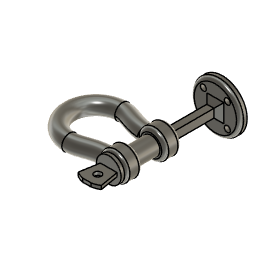
shackle v8 (Autodesk Fusion 360 design; units mm, degrees)
Autodesk Fusion 360 part; units mm, degrees
note: some values were not read from the file. Set by a fixed rule: which sketch regions a step uses.
sketch "Sketch1" plane through (0, 0, 0) normal (0, 0, 1) x (1, 0, 0)
  line L0 (0, 0) -> (0, -150) construction
  circle A0 centre (-62, -27) radius 37.5 construction
  line L1 (-62, -27) -> (-24.5, -27) construction
  line L2 (-62, -27) -> (-62, 10.5) construction
  spline S0 degree 5 poles (-62, 10.5) (-60.8613, 10.5) (-58.5805, 10.3966) (-55.1495, 9.9312) (-50.5421, 8.7566) (-44.6616, 6.7239) (-38.5882, 4.5603) (-32.2745, 2.6688) (-25.7346, 1.3084) (-19.0751, 0.4971) (-12.4478, 0.1204) (-7.3007, 0.0282) (-3.5865, 0.0051) (-1.1833, 0) (0, 0) knots 0 0 0 0 0 0 0.1 0.2 0.3 0.4 0.5 0.6 0.7 0.8 0.9 1 1 1 1 1 1
  line L3 (-6, 0) -> (6, 0)
  line L4 (-68, 10.5) -> (-56, 10.5)
  spline S1 degree 5 poles (-62, -64.5) (-60.8613, -64.5) (-58.5805, -64.3966) (-55.1495, -63.9312) (-50.5421, -62.7566) (-44.6616, -60.7239) (-38.5882, -58.5603) (-32.2745, -56.6688) (-25.7346, -55.3084) (-19.0751, -54.4971) (-12.4478, -54.1204) (-7.3007, -54.0282) (-3.5865, -54.0051) (-1.1833, -54) (0, -54) knots 0 0 0 0 0 0 0.1 0.2 0.3 0.4 0.5 0.6 0.7 0.8 0.9 1 1 1 1 1 1
  line L5 (-68, -64.5) -> (-56, -64.5)
  line L6 (-6, -54) -> (6, -54)
  arc A1 (-62, 10.5) -> (-62, -64.5) centre (-62, -27) ccw
  line L7 (-24.5, -27) -> (0, -27) construction
  line L8 (0, 0) -> (0, -27) construction
  point P0 (-33, 3)
  point P1 (-33, -57)
  dimension "d1" = 150
  dimension "d2" = 75
  constraint coincident L0.start S0.end
  constraint vertical L0
  constraint coincident A0.centre L1.start
  constraint coincident A0 L1.end
  constraint horizontal L1
  constraint coincident A0 L2.end
  constraint perpendicular L1 L2
  constraint midpoint L0.start L3
  constraint midpoint L2.end L4
  constraint tangent A0 L4
  constraint symmetric L0.start L1 S1.end
  constraint symmetric L1 L2.end S1.start
  constraint symmetric L1 P0 P1
  constraint symmetric L1 L3.start L6.start
  constraint symmetric L1 L3.end L6.end
  constraint symmetric L1 L4.start L5.start
  constraint symmetric L1 L4.end L5.end
  constraint coincident L0 L7.end
  constraint perpendicular L0 L7
  measures "d1" distance of L0.start L0.end
  measures "d2" diameter of A0
ref_plane "WorkPlane1" through (0, 0, 0) normal (1, 0, 0) x (0, 1, 0)
sketch "Sketch2" plane through (0, 0, 0) normal (1, 0, 0) x (0, 1, 0)
  circle A0 centre (0, 0) radius 11
  dimension "d4" = 22
  constraint coincident A0.centre origin
  measures "d4" diameter of A0
sweep "Sweep1" add profiles "Sketch2" path "Sketch1" along S1 A1 S0 section 1 makes body 1
sketch "Sketch3" plane through (0, 0, 0) normal (0, 1, 0) x (1, 0, 0)
  circle A0 centre (0, 0) radius 20
  circle A1 centre (0, 0) radius 12.5
  line L0 (5, -6) -> (-5, -6)
  line L1 (-5, -6) -> (-5, 6)
  line L2 (-5, 6) -> (5, 6)
  line L3 (5, 6) -> (5, -6)
  line L4 (5, -6) -> (-5, 6) construction
  line L5 (-5, -6) -> (5, 6) construction
  line L6 (-5.3, 6.3) -> (5.3, 6.3)
  line L7 (5.3, 6.3) -> (5.3, -6.3)
  line L8 (5.3, -6.3) -> (-5.3, -6.3)
  line L9 (-5.3, -6.3) -> (-5.3, 6.3)
  dimension "d11" = 40
  dimension "d16" = 25
  dimension "d70" = 10
  dimension "d71" = 12
  dimension "d72" = -0.3
  constraint coincident A0.centre A1.centre
  constraint concentric A0 A1
  constraint horizontal L0
  constraint perpendicular L0 L1
  constraint parallel L0 L2
  constraint parallel L1 L3
  constraint coincident L4 A0.centre
  constraint coincident L5 A0.centre
  measures "d11" diameter of A0
  measures "d16" diameter of A1
  measures "d70" distance of L1.end L2.end
  measures "d71" distance of L0.end L1.end
ref_plane "WorkPlane2" through (0, -27, 0) normal (0, 1, 0) x (0, 0, 1)
extrude "Extrude3" add sketch "Sketch3" along normal blind 12 and the other way blind 11 separate body contours A0 makes body 2
mirror "Mirror1" about plane through (0, -27, 0) normal (0, 1, 0) of bodies 2 makes body 3
combine "Combine1" operation add target body 1 tool bodies 2 3
extrude "Extrude4" cut sketch "Sketch3" along normal blind 16 and the other way blind 69 contours A1 | L0 L1 L2 L3 | L6 L7 L8 L9 bodies 1
fillet "Fillet1" radius 5 4 edges at (-18.6465, -43, -7.2323) (-18.6465, 12, 7.2323) (-18.6465, -11, -7.2323) (-18.6465, -66, 7.2323) on bodies 1
sketch "Sketch4" plane through (0, -66, 0) normal (0, -1, 0) x (1, 0, 0)
  circle A0 centre (0, 0) radius 12.5
  circle A1 centre (0, 0) radius 15
  circle A2 centre (0, 0) radius 12.5
  circle A3 centre (0, 0) radius 17.5
  line L0 (-17.5, 0.0312) -> (17.5, 0.0312) construction
  line L1 (17.3205, 2.5) -> (-17.3205, 2.5)
  line L2 (-17.3205, 2.5) -> (-17.3205, -2.5)
  line L3 (-17.3205, -2.5) -> (17.3205, -2.5)
  line L4 (17.3205, -2.5) -> (17.3205, 2.5)
  line L5 (17.3205, 2.5) -> (-17.3205, -2.5) construction
  line L6 (-17.3205, 2.5) -> (17.3205, -2.5) construction
  dimension "d35" = 25
  dimension "d36" = 35
  dimension "d39" = 5
  constraint coincident A0.centre A1.centre
  constraint coincident A3 L0.start
  constraint coincident A3 L0.end
  constraint horizontal L0
  constraint horizontal L1
  constraint perpendicular L1 L2
  constraint parallel L1 L3
  constraint parallel L2 L4
  constraint coincident A3 L1.start
  constraint coincident L5 A0.centre
  constraint coincident L6 A0.centre
  measures "d35" diameter of A2
  measures "d36" diameter of A3
  measures "d39" distance of L1.end L2.end
extrude "Extrude5" add sketch "Sketch4" along normal blind 5 bodies 1
extrude "Extrude6" add sketch "Sketch4" along normal blind 36 contours A0 A2 L1 L3 | A0 A1 A2 L1 L3 | A0 A1 A2 L1 L3 | A1 L1 L3 L4 | A1 L1 L2 L3 bodies 1
sketch "Sketch5" plane through (0, 0, 2.5) normal (0, 0, 1) x (-1, 0, 0)
  line L0 (-17.3205, 71) -> (17.3205, 71)
  line L1 (17.3205, 71) -> (17.3205, 102)
  line L2 (17.3205, 102) -> (-17.3205, 102)
  line L3 (-17.3205, 102) -> (-17.3205, 71)
  line L4 (0, 71) -> (0, 102) construction
  line L5 (11.7769, 71) -> (16.3887, 97.963)
  line L6 (-11.7769, 71) -> (-16.3887, 97.963)
  arc A0 (16.3887, 97.963) -> (-16.3887, 97.963) centre (0, 71.1337) ccw
  circle A1 centre (0, 86.5) radius 5
  dimension "d42" = 10
  constraint midpoint L0 L4.start
  constraint midpoint L2 L4.end
  constraint coincident L0 L5.start
  constraint symmetric L4 L5.start L6.start
  constraint symmetric L4 L5.end L6.end
  constraint midpoint L4 A1.centre
  measures "d42" diameter of A1
extrude "Extrude7" cut sketch "Sketch5" along normal up to surface (5 mm away) from surface at -5 contours L0 L2 L3 L6 A0 | L0 L1 L2 L5 A0 | A1 bodies 1
extrude "Extrude8" add sketch "Sketch3" along normal blind 12 and the other way up to surface (66 mm away) contours A1 | L0 L1 L2 L3 | L6 L7 L8 L9 bodies 1
extrude "Extrude12" cut sketch "Sketch3" along normal through all and the other way blind 40 contours L0 L1 L2 L3 | L6 L7 L8 L9 bodies 1
extrude "Extrude13" add sketch "Sketch3" along normal blind 90 and the other way blind 40 separate body contours L0 L1 L2 L3 makes body 4
sketch "Sketch8" plane through (0, 90, 0) normal (0, 1, 0) x (-1, 0, 0)
  line L0 (-5, -6) -> (5, -6)
  line L1 (5, -6) -> (5, 6)
  line L2 (5, 6) -> (-5, 6)
  line L3 (-5, 6) -> (-5, -6)
  circle A0 centre (0, 0) radius 35
  circle A1 centre (0, 0) radius 24 construction
  line L4 (0, 0) -> (24.7487, 24.7487) construction
  line L5 (0, 0) -> (35, 0) construction
  circle A2 centre (16.9706, 16.9706) radius 4.25
  circle A3 centre (-16.9706, 16.9706) radius 4.25
  circle A4 centre (-16.9706, -16.9706) radius 4.25
  circle A5 centre (16.9706, -16.9706) radius 4.25
  circle A6 centre (0, 0) radius 2
  dimension "d80" = 70
  dimension "d81" = 48
  dimension "d82" = 45
  dimension "d83" = 8.5
  dimension "d85" = 360
  dimension "d106" = 4
  constraint coincident A0.centre A1.centre
  constraint horizontal L5
  constraint coincident A0 L4.end
  constraint coincident A1 A2.centre
  constraint coincident L4 A2.centre
  measures "d80" diameter of A0
  measures "d81" diameter of A1
  measures "d82" angle of L4 L5
  measures "d83" diameter of A2
  measures "d106" diameter of A6
extrude "Extrude14" add sketch "Sketch8" against normal blind 10 contours A0 bodies 4
chamfer "Chamfer2" distance 7 angle 45 4 edges at (0, 80, 6) (5, 80, 0) (-5, 80, 0) (0, 80, -6) on bodies 4
fillet "Fillet3" radius 5 1 edges at (32.6315, 80, 12.6565) on bodies 4
sketch "Sketch9" plane through (0, 0, 0) normal (0, 0, 1) x (1, 0, 0)
box "BoxPrimitive2" add length 159.4331 width 179.6991 height 60 placed x (0, 1, 0) y (-1, 0, 0) z (0, 0, 1) at (55.4272, -112.9248, 0) separate body makes body 5
box "BoxPrimitive3" add length 193.3396 width 184.7162 height -50 placed x (0, 1, 0) y (-1, 0, 0) z (0, 0, 1) at (53.4506, -133.9959, 0) separate body makes body 6
extrude "Extrude15" cut sketch "Sketch8" against normal up to surface (130 mm away) contours A6 bodies 4
combine "Combine3" [suppressed]
combine "Combine2" [suppressed]
other "BoxPrimitive1"
hidden bodies 5 6
equation "d11 = 25 mm + 15 mm"
equation "d36 = 25 mm + 10 mm"
equation "d106 = 3.5 mm + 0.5 mm"
named bodies: "shackle", "stand", "cut upper", "cut lower"
